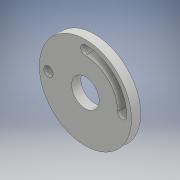
# Autodesk Inventor part: sprzeglo_02
Saved by Autodesk Inventor 2017 (Build 210142000, 142)
## iProperties
Created: 2021-05-20
Part Number: sprzeglo_02
Material: Generic
Document SubType Name: Modeling
Designer: majch
Density: 1 g/cm^3
Appearance: Default
Author: majch
Autodesk Inventor part; units mm, degrees
ref_plane "YZ Plane" through (0, 0, 0) normal (1, 0, 0) x (0, 1, 0)
ref_plane "XZ Plane" through (0, 0, 0) normal (0, 1, 0) x (-1, 0, 0)
ref_plane "XY Plane" through (0, 0, 0) normal (0, 0, 1) x (1, 0, 0)
sketch "Sketch1" plane through (0, 0, 0) normal (0, 1, 0) x (-1, 0, 0)
  circle A0 centre (0, 0) radius 25
  dimension "d0" = 50
  constraints: 1 centre point, 1 coincident
  measures "d0" diameter of A0
extrude "Extrusion1" add sketch "Sketch1" along normal blind 5
sketch "Sketch2" plane through (0, 5, 0) normal (0, 1, 0) x (1, 0, 0)
  circle A0 centre (0, 0) radius 7.5
  dimension "d3" = 15
  constraints: 1 centre point, 1 coincident
  measures "d3" diameter of A0
extrude "Extrusion2" cut sketch "Sketch2" against normal through all
sketch "Sketch4" plane through (0, 0, 0) normal (0, -1, 0) x (1, 0, 0)
  circle A0 centre (0, 0) radius 20 construction
  arc A1 (0, 22.5) -> (0, 17.5) centre (0, 20) ccw
  arc A2 (17.5, 0) -> (22.5, 0) centre (20, 0) ccw
  arc A3 (22.5, 0) -> (0, 22.5) centre (0, 0) ccw
  arc A4 (17.5, 0) -> (0, 17.5) centre (0, 0) ccw
  circle A5 centre (0, 0) radius 7.5 projected
  circle A6 centre (0, 0) radius 25 projected
  dimension "d9" = 5
  dimension "d10" = 5
  dimension "d11" = 90
  constraints: 10 point on circle, 5 centre point, 3 coincident
  measures "d9" diameter of A1
  measures "d10" diameter of A2
extrude "Extrusion3" cut sketch "Sketch4" against normal through all contours A3 A2 A4 A1
sketch "Sketch8" plane through (0, 0, 0) normal (0, -1, 0) x (1, 0, 0)
  circle A0 centre (0, 0) radius 20 construction
  arc A1 (22.5, 0) -> (0, 22.5) centre (0, 0) ccw projected
  arc A2 (17.5, 0) -> (22.5, 0) centre (20, 0) ccw projected
  arc A3 (17.5, 0) -> (0, 17.5) centre (0, 0) ccw projected
  arc A4 (0, 22.5) -> (0, 17.5) centre (0, 20) ccw projected
  circle A5 centre (0, 0) radius 7.5 projected
  circle A6 centre (0, 0) radius 25 projected
  arc A7 (17.5, 0) -> (0, 17.5) centre (0, 0) ccw projected
  circle A8 centre (0, 0) radius 25 projected
  circle A9 centre (-20, 0) radius 2.5
  dimension "d15" = 5
  constraints: 1 centre point, 2 other
  measures "d15" diameter of A9
extrude "Extrusion4" cut sketch "Sketch8" against normal through all contours A9
equation "\"kat_promienia\" = 30deg"
body "Solid1"
